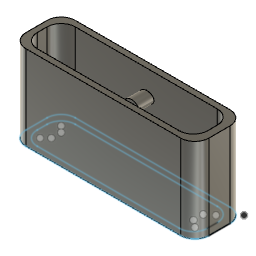
WatchStrapBit v5 (Autodesk Fusion 360 design; units mm, degrees)
Autodesk Fusion 360 part; units mm, degrees
note: some values were not read from the file. Set by a fixed rule: which sketch regions a step uses.
sketch "Sketch1" plane through (0, 0, 0) normal (0, 0, 1) x (1, 0, 0) in component "WatchStrapBit"
  line L0 (2, 0) -> (24, 0)
  line L1 (26, -2) -> (26, -5)
  line L2 (24, -7) -> (2, -7)
  line L3 (0, -5) -> (0, -2)
  line L4 (23, -0.8) -> (2.8, -0.8)
  line L5 (0.8, -2.8) -> (0.8, -4.2)
  line L6 (2.8, -6.2) -> (23, -6.2)
  line L7 (25, -4.2) -> (25, -2.8)
  arc A0 (25, -2.8) -> (23, -0.8) centre (23, -2.8) ccw
  arc A1 (23, -6.2) -> (25, -4.2) centre (23, -4.2) ccw
  arc A2 (2.8, -0.8) -> (0.8, -2.8) centre (2.8, -2.8) ccw
  arc A3 (0.8, -4.2) -> (2.8, -6.2) centre (2.8, -4.2) ccw
  arc A4 (2, 0) -> (0, -2) centre (2, -2) ccw
  arc A5 (0, -5) -> (2, -7) centre (2, -5) ccw
  arc A6 (24, -7) -> (26, -5) centre (24, -5) ccw
  arc A7 (26, -2) -> (24, 0) centre (24, -2) ccw
  point P0 (26, 0)
  dimension "d1" = 26
  dimension "d2" = 7
  dimension "d3" = 0.8
  dimension "d4" = 0.8
  dimension "d5" = 1
  dimension "d6" = 0.8
  dimension "d7" = 2
  constraint horizontal L0
  constraint vertical L1
  constraint horizontal L2
  constraint vertical L3
  constraint horizontal L4
  constraint vertical L5
  constraint horizontal L6
  constraint vertical L7
  constraint tangent L4 A0
  constraint tangent L7 A0
  constraint tangent L6 A1
  constraint tangent L7 A1
  constraint equal A0 A1
  constraint tangent L4 A2
  constraint tangent L5 A2
  constraint equal A0 A2
  constraint tangent L5 A3
  constraint tangent L6 A3
  constraint equal A0 A3
  constraint tangent L0 A4
  constraint tangent L3 A4
  constraint equal A0 A4
  constraint tangent L2 A5
  constraint tangent L3 A5
  constraint equal A0 A5
  constraint tangent L1 A6
  constraint tangent L2 A6
  constraint equal A0 A6
  constraint coincident P0 L0
  constraint coincident P0 L1
  constraint tangent L0 A7
  constraint tangent L1 A7
  constraint equal A0 A7
  measures "d1" distance of origin P0
  measures "d2" distance of L0 L2
  measures "d3" distance of L0 L4
  measures "d4" distance of L2 L6
  measures "d5" distance of L1 L7
  measures "d6" distance of L3 L5
  measures "d7" radius of A0
extrude "Extrude1" add sketch "Sketch1" along normal blind 12 in component "WatchStrapBit"
sketch "Sketch2" plane through (0, 0, 0) normal (0, 1, 0) x (-1, 0, 0) in component "WatchStrapBit"
  line L0 (-24, 0) -> (-2, 0)
  line L1 (-2, 0) -> (-2, 12)
  line L2 (-2, 12) -> (-24, 12)
  line L3 (-24, 12) -> (-24, 0)
  line L4 (-24, 0) -> (-2, 0)
  line L5 (-2, 12) -> (-24, 12)
  line L6 (0, 0) -> (-2, 0)
  line L7 (0, 12) -> (-2, 12)
  line L8 (0, 0) -> (0, 12)
  line L9 (-26, 0) -> (-26, 12)
  line L10 (-24, 0) -> (-26, 0)
  line L11 (-24, 12) -> (-26, 12)
  line L12 (0, 0) -> (-26, 0) construction
  line L13 (0, 12) -> (-26, 12) construction
  line L14 (-13, 0) -> (-13, 12) construction
  line L15 (-13, 6) -> (-13, 3.5)
  line L16 (-13, 6) -> (-13, 8.5)
  circle A0 centre (-13, 3.5) radius 0.75
  circle A1 centre (-13, 8.5) radius 0.75
  ellipse E0 centre (-13, 3.5) end of major axis (-13, 2.75) minor radius 1
  line L17 (-13, 4.25) -> (-13, 2.75)
  line L18 (-14, 3.5) -> (-12, 3.5)
  ellipse E1 centre (-13, 8.5) end of major axis (-13, 7.75) minor radius 1
  line L19 (-13, 9.25) -> (-13, 7.75)
  line L20 (-14, 8.5) -> (-12, 8.5)
  point P0 (-13, 0)
  point P1 (-13, 12)
  point P2 (-13, 6)
  dimension "d10" = 2.5
  dimension "d11" = 2.5
  dimension "d12" = 1.5
  dimension "d13" = 1.5
  dimension "d16" = 2
  dimension "d17" = 2
  constraint coincident L6.start L8.start
  constraint coincident L9.start L10.end
  constraint coincident L7.start L8.end
  constraint coincident L9.end L11.end
  constraint midpoint L12 P0
  constraint midpoint L13 P1
  constraint coincident P0 L14.start
  constraint coincident P1 L14.end
  constraint midpoint L14 P2
  constraint coincident P2 L15.start
  constraint perpendicular L12 L15
  constraint perpendicular L12 L16
  constraint coincident L15.end A0.centre
  constraint coincident L16.end A1.centre
  constraint coincident E0 L17.start
  constraint coincident E0 L17.end
  constraint coincident E0 L18.start
  constraint coincident E0 L18.end
  constraint concentric A0 E0
  constraint parallel L14 L17
  constraint coincident E1 L19.start
  constraint coincident E1 L19.end
  constraint coincident E1 L20.start
  constraint coincident E1 L20.end
  constraint concentric A1 E1
  measures "d10" distance of P2 L15.end
  measures "d11" distance of P2 L16.end
  measures "d12" diameter of A0
  measures "d13" diameter of A1
extrude "Extrude2" add sketch "Sketch2" against normal blind 3 contours L15 A0 L17 L18 | A0 E0 L18 | L15 A0 L17 L18 | A0 E0 L18 | A0 L17 L18 | A0 L17 L18 | A0 E0 L18 | A0 E0 L18 | L16 A1 L19 L20 | L16 A1 L19 L20 | A1 E1 L20 | A1 E1 L20 | A1 L19 L20 | A1 L19 L20 | A1 E1 L20 | A1 E1 L20 in component "WatchStrapBit"
component "WatchStrapBit" placed x (1, 0, 0) y (0, 1, 0) z (0, 0, 1) at (0, 0, 0)
equation "d4 = d3"
equation "d6 = d3"
named bodies: "WatchStrapBit"
